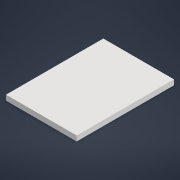
# Autodesk Inventor part: N_Bottom
Saved by Autodesk Inventor 2022 (Build 260153070, 153G)
## iProperties
Created: 2021-11-16
Part Number: N_Bottom
Material: Типовые
Document SubType Name: Modeling
Designer: kalugin_a
Density: 1 g/cm^3
Appearance: По умолчанию
Author: kalugin_a
Autodesk Inventor part; units mm, degrees
ref_plane "YZ Plane" through (0, 0, 0) normal (1, 0, 0) x (0, 1, 0)
ref_plane "XZ Plane" through (0, 0, 0) normal (0, 1, 0) x (-1, 0, 0)
ref_plane "XY Plane" through (0, 0, 0) normal (0, 0, 1) x (1, 0, 0)
sketch "Эскиз3" plane through (0, 0, 0) normal (0, 1, 0) x (-1, 0, 0)
  line L0 (0, 0) -> (218, 0)
  line L1 (218, 0) -> (218, -300)
  line L2 (218, -300) -> (0, -300)
  line L3 (0, -300) -> (0, 0)
  dimension "d4" = 218
  dimension "d5" = 300
  constraints: 8 end point, 2 parallel, 1 horizontal, 1 perpendicular
  measures "d4" distance of L1.end L2.end
  measures "d5" distance of L0.end L1.end
extrude "Выдавливание2" add sketch "Эскиз3" along normal blind 16
